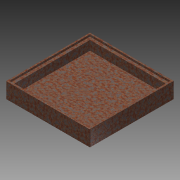
# Autodesk Inventor part: Propane Burner
Saved by Autodesk Inventor 2013 SP2 (Build 170200200, 200)
## iProperties
Created: 2014-05-29
Part Number: Propane Burner
Material: Steel
Document SubType Name: Modeling
Designer: rmclane
Density: 7.85 g/cm^3
Mass: 5958.17 g
Surface Area: 9072.97 cm^2
Volume: 759.002 cm^3
Author: rmclane
Autodesk Inventor part; units mm, degrees
ref_plane "YZ Plane" through (0, 0, 0) normal (1, 0, 0) x (0, 1, 0)
ref_plane "XZ Plane" through (0, 0, 0) normal (0, 1, 0) x (-1, 0, 0)
ref_plane "XY Plane" through (0, 0, 0) normal (0, 0, 1) x (1, 0, 0)
sketch "Sketch1" plane through (0, 0, 0) normal (0, 1, 0) x (-1, 0, 0)
  line L0 (-419.9992, 0) -> (419.9992, 0) projected
  line L1 (0, -419.9992) -> (0, 419.9992) projected
  line L2 (-299.9994, 299.9994) -> (299.9994, 299.9994)
  line L3 (299.9994, 299.9994) -> (299.9994, -299.9994)
  line L4 (299.9994, -299.9994) -> (-299.9994, -299.9994)
  line L5 (-299.9994, -299.9994) -> (-299.9994, 299.9994)
  line L6 (419.9992, 0) -> (-419.9992, 0) projected
  line L7 (0, -419.9992) -> (0, 419.9992) projected
  line L8 (287.2994, -287.2994) -> (-287.2994, -287.2994)
  line L9 (-287.2994, -287.2994) -> (-287.2994, 287.2994)
  line L10 (-287.2994, 287.2994) -> (287.2994, 287.2994)
  line L11 (287.2994, 287.2994) -> (287.2994, -287.2994)
  point P0 (0, 0)
  dimension "d0" = 599.9988
  dimension "d2" = 599.9988
  dimension "d3" = 574.5988
  dimension "d4" = 574.5988
  constraints: 16 end point, 4 parallel, 2 horizontal, 2 perpendicular, 4 other
  measures "d0" distance between parallel lines of L3 L5
  measures "d2" distance between parallel lines of L2 L4
  measures "d3" distance between parallel lines of L9 L11
  measures "d4" distance between parallel lines of L10 L8
extrude "Extrusion1" add sketch "Sketch1" against normal blind 1.5875 contours L5 L2 L1 L10 L9 L0 | L0 L9 L8 L1 L4 L5 | L1 L8 L11 L0 L3 L4 | L2 L3 L0 L11 L10 L1
sketch "Sketch2" plane through (0, -1.5875, 0) normal (0, -1, 0) x (1, 0, 0)
  line L0 (299.9994, 299.9994) -> (-299.9994, 299.9994) projected
  line L1 (-299.9994, 299.9994) -> (-299.9994, -299.9994) projected
  line L2 (-299.9994, -299.9994) -> (299.9994, -299.9994) projected
  line L3 (299.9994, -299.9994) -> (299.9994, 299.9994) projected
  line L4 (-287.2994, -287.2994) -> (-287.2994, 287.2994) projected
  line L5 (-287.2994, 287.2994) -> (287.2994, 287.2994) projected
  line L6 (287.2994, 287.2994) -> (287.2994, -287.2994) projected
  line L7 (287.2994, -287.2994) -> (-287.2994, -287.2994) projected
  line L8 (299.9994, 299.9994) -> (-299.9994, 299.9994) projected
  line L9 (-299.9994, 299.9994) -> (-299.9994, -299.9994) projected
  line L10 (-299.9994, -299.9994) -> (299.9994, -299.9994) projected
  line L11 (299.9994, -299.9994) -> (299.9994, 299.9994) projected
  line L12 (0, -419.9992) -> (0, 419.9992) projected
  line L13 (-419.9992, 0) -> (419.9992, 0) projected
  line L14 (-298.4119, 298.4119) -> (298.4119, 298.4119)
  line L15 (298.4119, 298.4119) -> (298.4119, -298.4119)
  line L16 (298.4119, -298.4119) -> (-298.4119, -298.4119)
  line L17 (-298.4119, -298.4119) -> (-298.4119, 298.4119)
  point P0 (0, 0)
  dimension "d7" = 1.5875
  dimension "d8" = 1.5875
  constraints: 8 end point, 2 parallel, 1 horizontal, 1 perpendicular, 2 other
  measures "d7" distance between parallel lines of L0 L14
  measures "d8" distance between parallel lines of L1 L17
extrude "Extrusion2" add sketch "Sketch2" along normal blind 111.125 contours L3 L13 L15 L14 L12 L0 | L12 L14 L17 L13 L1 L0 | L3 L2 L12 L16 L15 L13 | L13 L17 L16 L12 L2 L1
sketch "Sketch3" plane through (0, -112.7125, 0) normal (0, -1, 0) x (1, 0, 0)
  line L0 (-419.9992, 0) -> (419.9992, 0) projected
  line L1 (0, -419.9992) -> (0, 419.9992) projected
  line L2 (-299.9994, 299.9994) -> (299.9994, 299.9994)
  line L3 (299.9994, 299.9994) -> (299.9994, -299.9994)
  line L4 (299.9994, -299.9994) -> (-299.9994, -299.9994)
  line L5 (-299.9994, -299.9994) -> (-299.9994, 299.9994)
  point P0 (0, 0)
  constraints: 8 end point, 2 parallel, 1 horizontal, 1 perpendicular
extrude "Extrusion3" add sketch "Sketch3" along normal blind 1.5875
ref_plane "Work Plane1" through (0, -25.4, 0) normal (0, 1, 0) x (1, 0, 0)
sketch "Sketch4" plane through (0, -25.4, 0) normal (0, 1, 0) x (1, 0, 0)
  line L0 (298.4119, -298.4119) -> (298.4119, 298.4119) projected
  line L1 (298.4119, 298.4119) -> (-298.4119, 298.4119) projected
  line L2 (-298.4119, 298.4119) -> (-298.4119, -298.4119) projected
  line L3 (-298.4119, -298.4119) -> (298.4119, -298.4119) projected
  line L4 (-299.9994, -299.9994) -> (-299.9994, 299.9994) projected
  line L5 (-299.9994, 299.9994) -> (299.9994, 299.9994) projected
  line L6 (299.9994, 299.9994) -> (299.9994, -299.9994) projected
  line L7 (299.9994, -299.9994) -> (-299.9994, -299.9994) projected
  line L8 (-277.7617, 277.7744) -> (277.7617, 277.7744)
  line L9 (277.7617, 277.7744) -> (277.7617, -277.7744)
  line L10 (277.7617, -277.7744) -> (-277.7617, -277.7744)
  line L11 (-277.7617, -277.7744) -> (-277.7617, 277.7744)
  line L12 (419.9992, 0) -> (-419.9992, 0) projected
  line L13 (0, 419.9992) -> (0, -419.9992) projected
  point P0 (0, 0)
  dimension "d14" = 20.6375
  dimension "d15" = 20.6502
  dimension "d74" = 44.45
  dimension "d75" = 38.1
  dimension "d76" = 31.75
  constraints: 8 end point, 2 parallel, 1 horizontal, 1 perpendicular, 2 other
  measures "d14" distance between parallel lines of L1 L8
  measures "d15" distance between parallel lines of L2 L11
extrude "Extrusion4" add sketch "Sketch4" against normal blind 1.5875 contours L3 L13 L10 L9 L12 L0 | L12 L9 L8 L13 L1 L0 | L3 L2 L12 L11 L10 L13 | L13 L8 L11 L12 L2 L1
fillet "Fillet1" radius 3.175 12 edges at (0, 0, 299.9994) (0, -114.3, 299.9994) (299.9994, -57.15, 299.9994) (299.9994, -114.3, 0) (299.9994, 0, 0) (299.9994, -57.15, -299.9994) (0, 0, -299.9994) (-299.9994, 0, 0) (-299.9994, -57.15, 299.9994) (0, -114.3, -299.9994) (-299.9994, -57.15, -299.9994) (-299.9994, -114.3, 0)
sketch "Sketch6" plane through (-298.4119, -112.7125, -298.4119) normal (0, 0, 1) x (1, 0, 0)
  circle A0 centre (298.4119, 42.8625) radius 15.875 projected
  circle A1 centre (298.4119, 42.8625) radius 15.875
  circle A2 centre (298.4119, 42.8625) radius 12.7
  point P0 (298.4119, 112.7125)
  dimension "d83" = 25.4
  constraints: 2 centre point, 2 coincident, 1 concentric
  measures "d83" diameter of A2
sketch "Sketch7" plane through (299.9994, -111.125, 296.8244) normal (1, 0, 0) x (0, 0, -1)
  line L0 (593.6488, 111.125) -> (0, 111.125) projected
  line L1 (296.8244, -26.035) -> (296.8244, 133.985) projected
  circle A0 centre (55.5752, 95.25) radius 3.175
  line L2 (-1.5875, 109.5375) -> (-1.5875, 85.725) projected
  line L3 (-3.175, 107.95) -> (-3.175, 0) projected
  circle A1 centre (538.0736, 95.25) radius 3.175
  point P0 (296.8244, 111.125)
  dimension "d91" = 6.35
  dimension "d95" = 58.7502
  dimension "d96" = 15.875
  constraints: 2 centre point, 1 symmetric about line, 1 other
  measures "d91" diameter of A0
  measures "d95" distance from line of L3 A0.centre
  measures "d96" distance from line of L0 A0.centre
body "Solid1"
